Autodesk Inventor part; units mm, degrees
(part 2 of 3)
  arc A175 (-46.3689, 72.515) -> (-46.5311, 72.3209) centre (-45.3427, 71.4927) ccw
  line L41 (-46.5311, 72.3209) -> (-46.5959, 72.2278)
  line L42 (-46.5959, 72.2278) -> (-45.9786, 71.6449)
  line L43 (-45.9786, 71.6449) -> (-45.3612, 71.062)
  line L44 (-45.3612, 71.062) -> (-45.235, 71.2144)
  arc A176 (-44.7219, 71.7621) -> (-45.235, 71.2144) centre (-40.503, 67.2955) ccw
  arc A177 (-44.1577, 72.2287) -> (-44.7219, 71.7621) centre (-40.8999, 67.7158) ccw
  arc A178 (-43.5459, 72.611) -> (-44.1577, 72.2287) centre (-40.9969, 67.8501) ccw
  arc A179 (-42.8903, 72.907) -> (-43.5459, 72.611) centre (-41.0276, 67.9074) ccw
  arc A180 (-41.2076, 73.2541) -> (-42.8903, 72.907) centre (-40.9253, 67.6328) ccw
  arc A181 (-39.5165, 73.0714) -> (-41.2076, 73.2541) centre (-40.9361, 67.8491) ccw
  arc A182 (-37.9591, 72.3712) -> (-39.5165, 73.0714) centre (-40.9482, 67.8045) ccw
  arc A183 (-36.6652, 71.2147) -> (-37.9591, 72.3712) centre (-41.1435, 67.5061) ccw
  line L45 (-36.6652, 71.2147) -> (-36.5393, 71.0627)
  line L46 (-36.5393, 71.0627) -> (-35.9223, 71.6459)
  line L47 (-35.9223, 71.6459) -> (-35.3053, 72.2292)
  line L48 (-35.3053, 72.2292) -> (-35.3698, 72.3216)
  arc A184 (-35.3698, 72.3216) -> (-35.4148, 72.3777) centre (-35.8109, 72.0138) ccw
  arc A185 (-35.4148, 72.3777) -> (-35.5379, 72.51) centre (-46.5034, 62.1891) ccw
  arc A186 (-35.5379, 72.51) -> (-35.6869, 72.6659) centre (-45.6213, 63.0194) ccw
  arc A187 (-35.6869, 72.6659) -> (-35.8513, 72.8332) centre (-49.5707, 59.1844) ccw
  arc A188 (-35.8513, 72.8332) -> (-36.3178, 73.2672) centre (-41.6997, 67.0149) ccw
  arc A189 (-36.3178, 73.2672) -> (-36.7902, 73.6373) centre (-40.5561, 68.3435) ccw
  arc A190 (-36.7902, 73.6373) -> (-37.294, 73.9616) centre (-40.5426, 68.3625) ccw
  arc A191 (-37.294, 73.9616) -> (-37.8545, 74.2582) centre (-41.3698, 66.9368) ccw
  arc A192 (-37.8545, 74.2582) -> (-38.4115, 74.496) centre (-40.8225, 68.0766) ccw
  arc A193 (-38.4115, 74.496) -> (-38.9986, 74.689) centre (-41.0253, 67.5365) ccw
  arc A194 (-38.9986, 74.689) -> (-39.6005, 74.8329) centre (-41.0306, 67.518) ccw
  arc A195 (-39.6005, 74.8329) -> (-40.2018, 74.9233) centre (-40.9339, 68.0123) ccw
  arc A196 (-40.2018, 74.9233) -> (-40.5238, 74.9445) centre (-40.629, 70.891) ccw
  arc A197 (-40.5238, 74.9445) -> (-40.9902, 74.9502) centre (-40.9642, 57.9715) ccw
  arc A198 (-40.9902, 74.9502) -> (-41.4524, 74.9433) centre (-40.9639, 57.7224) ccw
  arc A199 (-41.4524, 74.9433) -> (-41.7507, 74.9209) centre (-41.3609, 71.7201) ccw
  arc A200 (-41.2579, 72.1952) -> (-42.0544, 72.0566) centre (-40.7232, 66.7647) ccw
  arc A201 (-42.0544, 72.0566) -> (-42.777, 71.8059) centre (-40.9868, 67.8125) ccw
  arc A202 (-42.777, 71.8059) -> (-43.4305, 71.4395) centre (-41.064, 67.9846) ccw
  arc A203 (-43.4305, 71.4395) -> (-44.0216, 70.9563) centre (-40.8808, 67.7173) ccw
  arc A204 (-44.0216, 70.9563) -> (-44.2114, 70.7646) centre (-39.4249, 66.2158) ccw
  arc A205 (-44.2114, 70.7646) -> (-44.3924, 70.5661) centre (-39.5049, 66.2919) ccw
  arc A206 (-44.3924, 70.5661) -> (-44.5501, 70.3821) centre (-35.0685, 62.4121) ccw
  arc A207 (-44.5501, 70.3821) -> (-44.5689, 70.3304) centre (-44.4886, 70.3304) ccw
  arc A208 (-44.5689, 70.3304) -> (-44.5593, 70.3082) centre (-44.5383, 70.3304) ccw
  arc A209 (-44.5593, 70.3082) -> (-43.965, 69.7486) centre (1428.2979, 1633.9609) ccw
  arc A210 (-43.965, 69.7486) -> (-43.3785, 69.197) centre (709.8736, 870.6675) ccw
  arc A211 (-43.3785, 69.197) -> (-43.337, 69.1709) centre (-43.2914, 69.2897) ccw
  arc A212 (-43.337, 69.1709) -> (-43.3227, 69.1742) centre (-43.3323, 69.1832) ccw
  arc A213 (-43.3227, 69.1742) -> (-43.2796, 69.2215) centre (-44.5899, 70.3724) ccw
  arc A214 (-43.2796, 69.2215) -> (-43.2296, 69.2821) centre (-44.2462, 70.0705) ccw
  arc A215 (-43.2296, 69.2821) -> (-43.1747, 69.3557) centre (-45.1202, 70.7483) ccw
  arc A216 (-42.8453, 69.7346) -> (-43.1747, 69.3557) centre (-41.0102, 67.8065) ccw
  arc A217 (-42.4468, 70.05) -> (-42.8453, 69.7346) centre (-40.9199, 67.7116) ccw
  arc A218 (-41.9954, 70.2896) -> (-42.4468, 70.05) centre (-40.9017, 67.6837) ccw
  arc A219 (-41.5087, 70.4437) -> (-41.9954, 70.2896) centre (-40.9069, 67.6961) ccw
  arc A220 (-41.2232, 70.4813) -> (-41.5087, 70.4437) centre (-41.1431, 68.7745) ccw
  arc A221 (-40.8534, 70.4837) -> (-41.2232, 70.4813) centre (-41.0092, 65.9221) ccw
  arc A222 (-40.4843, 70.4561) -> (-40.8534, 70.4837) centre (-41.0093, 65.9186) ccw
  arc A223 (-40.2008, 70.399) -> (-40.4843, 70.4561) centre (-40.6834, 68.7357) ccw
  arc A224 (-39.7681, 70.2293) -> (-40.2008, 70.399) centre (-40.9106, 67.9526) ccw
  arc A225 (-39.3522, 69.9772) -> (-39.7681, 70.2293) centre (-41.1362, 67.5029) ccw
  arc A226 (-38.983, 69.6632) -> (-39.3522, 69.9772) centre (-41.1244, 67.5193) ccw
  arc A227 (-38.6894, 69.3092) -> (-38.983, 69.6632) centre (-40.7215, 67.9227) ccw
  arc A228 (-38.6894, 69.3092) -> (-38.6489, 69.2532) centre (-37.6233, 70.0366) ccw
  arc A229 (-38.6489, 69.2532) -> (-38.6109, 69.2074) centre (-38.0844, 69.6844) ccw
  arc A230 (-38.6109, 69.2074) -> (-38.5781, 69.1735) centre (-38.075, 69.6929) ccw
  arc A231 (-38.5781, 69.1735) -> (-38.5639, 69.1706) centre (-38.5687, 69.1832) ccw
  arc A232 (-38.5639, 69.1706) -> (-38.5237, 69.1957) centre (-38.6075, 69.285) ccw
  arc A233 (-38.5237, 69.1957) -> (-37.9358, 69.7477) centre (-850.002, 934.1296) ccw
  arc A234 (-37.9358, 69.7477) -> (-37.3402, 70.3074) centre (-1609.827, 1742.9056) ccw
  arc A235 (-37.3402, 70.3074) -> (-37.3309, 70.3289) centre (-37.3604, 70.3289) ccw
  arc A236 (-37.3309, 70.3289) -> (-37.3338, 70.3377) centre (-37.3457, 70.3289) ccw
  arc A237 (-37.3338, 70.3377) -> (-37.376, 70.3946) centre (-47.3292, 62.9655) ccw
  arc A238 (-37.376, 70.3946) -> (-37.4256, 70.4597) centre (-40.8459, 67.8046) ccw
  arc A239 (-37.4256, 70.4597) -> (-37.4844, 70.5345) centre (-43.6707, 65.6119) ccw
  arc A240 (-37.4844, 70.5345) -> (-37.79, 70.8727) centre (-40.3313, 68.2691) ccw
  arc A241 (-37.79, 70.8727) -> (-38.1676, 71.2088) centre (-41.6249, 66.9438) ccw
  arc A242 (-38.1676, 71.2088) -> (-38.5756, 71.5096) centre (-41.641, 66.9241) ccw
  arc A243 (-38.5756, 71.5096) -> (-38.9731, 71.7413) centre (-40.6602, 68.3913) ccw
  arc A244 (-38.9731, 71.7413) -> (-39.2289, 71.8543) centre (-40.2179, 69.2696) ccw
  arc A245 (-39.2289, 71.8543) -> (-39.5614, 71.9719) centre (-41.6999, 65.3962) ccw
  arc A246 (-39.5614, 71.9719) -> (-39.9011, 72.0729) centre (-41.7094, 65.3668) ccw
  arc A247 (-39.9011, 72.0729) -> (-40.1799, 72.1338) centre (-40.6703, 69.2201) ccw
  arc A248 (-40.1799, 72.1338) -> (-40.4304, 72.1665) centre (-40.7514, 68.7389) ccw
  arc A249 (-40.4304, 72.1665) -> (-40.7499, 72.1906) centre (-41.2496, 63.417) ccw
  arc A250 (-40.7499, 72.1906) -> (-41.0583, 72.2028) centre (-41.2542, 63.3377) ccw
  arc A251 (-41.0583, 72.2028) -> (-41.2579, 72.1952) centre (-41.095, 70.5405) ccw
  arc A252 (-41.3041, 69.3977) -> (-41.7203, 69.2048) centre (-40.9224, 68.0282) ccw
  arc A253 (-41.7203, 69.2048) -> (-42.057, 68.8883) centre (-40.8992, 67.9939) ccw
  arc A254 (-42.057, 68.8883) -> (-42.2759, 68.4855) centre (-40.9189, 68.0091) ccw
  arc A255 (-42.2759, 68.4855) -> (-42.351, 68.0425) centre (-41.0214, 68.0451) ccw
  arc A256 (-42.351, 68.0425) -> (-42.2073, 67.4314) centre (-40.9678, 68.0452) ccw
  arc A257 (-42.2073, 67.4314) -> (-41.8076, 66.9404) centre (-40.9266, 68.0656) ccw
  arc A258 (-41.8076, 66.9404) -> (-41.2375, 66.6724) centre (-40.937, 68.0524) ccw
  arc A259 (-41.2375, 66.6724) -> (-40.6171, 66.6849) centre (-40.9535, 67.9765) ccw
  arc A260 (-40.6171, 66.6849) -> (-40.2585, 66.8282) centre (-41.0066, 68.1804) ccw
  arc A261 (-40.2585, 66.8282) -> (-39.9614, 67.0519) centre (-40.9034, 67.9939) ccw
  arc A262 (-39.9614, 67.0519) -> (-39.7377, 67.3489) centre (-40.9034, 67.9939) ccw
  arc A263 (-39.7377, 67.3489) -> (-39.5945, 67.7075) centre (-41.0899, 68.0971) ccw
  arc A264 (-39.5945, 67.7075) -> (-39.5827, 68.335) centre (-40.8932, 68.0458) ccw
  arc A265 (-39.5827, 68.335) -> (-39.8564, 68.9075) centre (-40.949, 68.0335) ccw
  arc A266 (-39.8564, 68.9075) -> (-40.3572, 69.3039) centre (-40.9658, 68.02) ccw
  arc A267 (-40.3572, 69.3039) -> (-40.9795, 69.439) centre (-40.9587, 68.0351) ccw
  arc A268 (-40.9795, 69.439) -> (-41.0608, 69.4352) centre (-40.9611, 68.1934) ccw
  arc A269 (-41.0608, 69.4352) -> (-41.1516, 69.4257) centre (-40.904, 67.4834) ccw
  arc A270 (-41.1516, 69.4257) -> (-41.2378, 69.4127) centre (-40.9176, 67.5898) ccw
  arc A271 (-41.2378, 69.4127) -> (-41.3041, 69.3977) centre (-41.1176, 68.7282) ccw
  arc A272 (-54.2587, 71.8195) -> (-55.2164, 71.6633) centre (-53.721, 65.5053) ccw
  arc A273 (-55.2164, 71.6633) -> (-56.1281, 71.3638) centre (-53.7854, 65.7705) ccw
  arc A274 (-56.1281, 71.3638) -> (-56.9803, 70.9245) centre (-53.7898, 65.7811) ccw
  arc A275 (-56.9803, 70.9245) -> (-57.761, 70.3525) centre (-53.6689, 65.5862) ccw
  arc A276 (-57.761, 70.3525) -> (-57.9303, 70.1998) centre (-54.7143, 66.8038) ccw
  arc A277 (-57.9303, 70.1998) -> (-58.1244, 70.0106) centre (-51.5447, 63.4568) ccw
  arc A278 (-58.1244, 70.0106) -> (-58.3037, 69.8254) centre (-51.7023, 63.6139) ccw
  arc A279 (-58.3037, 69.8254) -> (-58.4189, 69.6921) centre (-56.7958, 68.4066) ccw
  line L49 (-58.4189, 69.6921) -> (-58.4764, 69.6194)
  line L50 (-58.4764, 69.6194) -> (-58.0951, 69.2684)
  line L51 (-58.0951, 69.2684) -> (-57.7138, 68.9174)
  line L52 (-57.7138, 68.9174) -> (-57.6118, 69.0338)
  arc A280 (-57.0139, 69.616) -> (-57.6118, 69.0338) centre (-53.6679, 65.5813) ccw
  arc A281 (-56.3308, 70.0963) -> (-57.0139, 69.616) centre (-53.6618, 65.5739) ccw
  arc A282 (-55.5869, 70.4582) -> (-56.3308, 70.0963) centre (-53.7111, 65.6576) ccw
  arc A283 (-54.8079, 70.6887) -> (-55.5869, 70.4582) centre (-53.8421, 65.9928) ccw
  arc A284 (-54.2943, 70.7669) -> (-54.8079, 70.6887) centre (-53.7974, 65.7752) ccw
  arc A285 (-53.7678, 70.793) -> (-54.2943, 70.7669) centre (-53.7678, 65.4777) ccw
  arc A286 (-53.2413, 70.7669) -> (-53.7678, 70.793) centre (-53.7678, 65.4777) ccw
  arc A287 (-52.7277, 70.6887) -> (-53.2413, 70.7669) centre (-53.7382, 65.7752) ccw
  arc A288 (-51.9486, 70.4585) -> (-52.7277, 70.6887) centre (-53.6976, 65.9726) ccw
  arc A289 (-51.2067, 70.0979) -> (-51.9486, 70.4585) centre (-53.8074, 65.6909) ccw
  arc A290 (-50.5247, 69.6182) -> (-51.2067, 70.0979) centre (-53.8645, 65.5942) ccw
  arc A291 (-49.9239, 69.034) -> (-50.5247, 69.6182) centre (-53.9323, 65.5125) ccw
  line L53 (-49.9239, 69.034) -> (-49.8218, 68.9178)
  line L54 (-49.8218, 68.9178) -> (-49.4403, 69.2684)
  line L55 (-49.4403, 69.2684) -> (-49.0588, 69.619)
  line L56 (-49.0588, 69.619) -> (-49.1187, 69.6961)
  arc A292 (-49.1187, 69.6961) -> (-49.2435, 69.8387) centre (-50.3783, 68.7188) ccw
  arc A293 (-49.2435, 69.8387) -> (-49.4908, 70.0838) centre (-60.4502, 58.7794) ccw
  arc A294 (-49.4908, 70.0838) -> (-49.7488, 70.3278) centre (-59.4752, 59.7852) ccw
  arc A295 (-49.7488, 70.3278) -> (-49.9351, 70.4876) centre (-52.0641, 67.8182) ccw
  arc A296 (-49.9351, 70.4876) -> (-50.698, 71.0097) centre (-53.8793, 65.5422) ccw
  arc A297 (-50.698, 71.0097) -> (-51.5212, 71.4089) centre (-53.7491, 65.766) ccw
  arc A298 (-51.5212, 71.4089) -> (-52.3959, 71.6801) centre (-53.7544, 65.7527) ccw
  arc A299 (-52.3959, 71.6801) -> (-53.3127, 71.8212) centre (-53.8245, 65.4466) ccw
  arc A300 (-53.3127, 71.8212) -> (-53.5357, 71.8337) centre (-53.6841, 67.195) ccw
  arc A301 (-53.5357, 71.8337) -> (-53.7872, 71.8375) centre (-53.7737, 64.3958) ccw
  arc A302 (-53.7872, 71.8375) -> (-54.0379, 71.8328) centre (-53.7737, 64.4287) ccw
  arc A303 (-54.0379, 71.8328) -> (-54.2587, 71.8195) centre (-53.8779, 67.3479) ccw
  arc A304 (-54.2587, 70.1206) -> (-54.8466, 70.011) centre (-53.685, 65.4098) ccw
  arc A305 (-54.8466, 70.011) -> (-55.4044, 69.8298) centre (-53.7721, 65.755) ccw
  arc A306 (-55.4044, 69.8298) -> (-55.9344, 69.5753) centre (-53.7639, 65.7344) ccw
  arc A307 (-55.9344, 69.5753) -> (-56.4394, 69.2471) centre (-53.5452, 65.3475) ccw
  arc A308 (-56.4394, 69.2471) -> (-56.6021, 69.1131) centre (-55.1906, 67.5645) ccw
  arc A309 (-56.6021, 69.1131) -> (-56.8494, 68.8817) centre (-47.9272, 59.5958) ccw
  arc A310 (-56.8494, 68.8817) -> (-57.0896, 68.6458) centre (-46.1793, 57.7765) ccw
  arc A311 (-57.0896, 68.6458) -> (-57.189, 68.5268) centre (-56.4605, 68.0191) ccw
  line L57 (-57.189, 68.5268) -> (-57.2288, 68.4697)
  line L58 (-57.2288, 68.4697) -> (-56.8503, 68.1124)
  line L59 (-56.8503, 68.1124) -> (-56.4719, 67.7551)
  line L60 (-56.4719, 67.7551) -> (-56.3945, 67.8485)
  arc A312 (-56.08, 68.1842) -> (-56.3945, 67.8485) centre (-53.4938, 65.4462) ccw
  arc A313 (-55.7342, 68.4703) -> (-56.08, 68.1842) centre (-53.7371, 65.7039) ccw
  arc A314 (-55.3591, 68.7046) -> (-55.7342, 68.4703) centre (-53.7966, 65.7862) ccw
  arc A315 (-54.9572, 68.886) -> (-55.3591, 68.7046) centre (-53.8154, 65.8213) ccw
  arc A316 (-53.9257, 69.0988) -> (-54.9572, 68.886) centre (-53.7527, 65.653) ccw
  arc A317 (-52.8891, 68.9868) -> (-53.9257, 69.0988) centre (-53.7593, 65.7856) ccw
  arc A318 (-51.9344, 68.5576) -> (-52.8891, 68.9868) centre (-53.7667, 65.7582) ccw
  arc A319 (-51.1412, 67.8487) -> (-51.9344, 68.5576) centre (-53.8865, 65.5753) ccw
  line L61 (-51.1412, 67.8487) -> (-51.064, 67.7555)
  line L62 (-51.064, 67.7555) -> (-50.6858, 68.113)
  line L63 (-50.6858, 68.113) -> (-50.3077, 68.4706)
  line L64 (-50.3077, 68.4706) -> (-50.3472, 68.5272)
  arc A320 (-50.3472, 68.5272) -> (-50.3748, 68.5616) centre (-50.6176, 68.3385) ccw
  arc A321 (-50.3748, 68.5616) -> (-50.4502, 68.6427) centre (-57.1721, 62.316) ccw
  arc A322 (-50.4502, 68.6427) -> (-50.5416, 68.7383) centre (-56.6313, 62.825) ccw
  arc A323 (-50.5416, 68.7383) -> (-50.6423, 68.8408) centre (-59.0523, 60.4741) ccw
  arc A324 (-50.6423, 68.8408) -> (-50.9283, 69.1069) centre (-54.2274, 65.2742) ccw
  arc A325 (-50.9283, 69.1069) -> (-51.2179, 69.3337) centre (-53.5264, 66.0886) ccw
  arc A326 (-51.2179, 69.3337) -> (-51.5267, 69.5325) centre (-53.5181, 66.1003) ccw
  arc A327 (-51.5267, 69.5325) -> (-51.8703, 69.7143) centre (-54.0251, 65.2263) ccw
  arc A328 (-51.8703, 69.7143) -> (-52.2117, 69.8601) centre (-53.6897, 65.9251) ccw
  arc A329 (-52.2117, 69.8601) -> (-52.5716, 69.9784) centre (-53.814, 65.594) ccw
  arc A330 (-52.5716, 69.9784) -> (-52.9406, 70.0666) centre (-53.8172, 65.5826) ccw
  arc A331 (-52.9406, 70.0666) -> (-53.3092, 70.1221) centre (-53.758, 65.8856) ccw
  arc A332 (-53.3092, 70.1221) -> (-53.5066, 70.1351) centre (-53.571, 67.6502) ccw
  arc A333 (-53.5066, 70.1351) -> (-53.7925, 70.1386) centre (-53.7766, 59.7306) ccw
  arc A334 (-53.7925, 70.1386) -> (-54.0758, 70.1343) centre (-53.7763, 59.5779) ccw
  arc A335 (-54.0758, 70.1343) -> (-54.2587, 70.1206) centre (-54.0197, 68.1585) ccw
  arc A336 (-53.9566, 68.4497) -> (-54.4448, 68.3648) centre (-53.6288, 65.1208) ccw
  arc A337 (-54.4448, 68.3648) -> (-54.8878, 68.2111) centre (-53.7904, 65.7631) ccw
  arc A338 (-54.8878, 68.2111) -> (-55.2884, 67.9865) centre (-53.8377, 65.8687) ccw
  arc A339 (-55.2884, 67.9865) -> (-55.6507, 67.6903) centre (-53.7254, 65.7048) ccw
  arc A340 (-55.6507, 67.6903) -> (-55.7671, 67.5728) centre (-52.8329, 64.7844) ccw
  arc A341 (-55.7671, 67.5728) -> (-55.878, 67.4511) centre (-52.882, 64.831) ccw
  arc A342 (-55.878, 67.4511) -> (-55.9747, 67.3383) centre (-50.1625, 62.4527) ccw
  arc A343 (-55.9747, 67.3383) -> (-55.9862, 67.3066) centre (-55.937, 67.3066) ccw
  arc A344 (-55.9862, 67.3066) -> (-55.9803, 67.293) centre (-55.9675, 67.3066) ccw
  arc A345 (-55.9803, 67.293) -> (-55.616, 66.95) centre (846.8811, 1025.8121) ccw
  arc A346 (-55.616, 66.95) -> (-55.2565, 66.6118) centre (406.487, 557.9133) ccw
  arc A347 (-55.2565, 66.6118) -> (-55.2311, 66.5959) centre (-55.2031, 66.6687) ccw
  arc A348 (-55.2311, 66.5959) -> (-55.2223, 66.5979) centre (-55.2282, 66.6034) ccw
  arc A349 (-55.2223, 66.5979) -> (-55.1959, 66.6269) centre (-55.9991, 67.3324) ccw
  arc A350 (-55.1959, 66.6269) -> (-55.1652, 66.664) centre (-55.7884, 67.1473) ccw
  arc A351 (-55.1652, 66.664) -> (-55.1316, 66.7092) centre (-56.3242, 67.5628) ccw
  arc A352 (-54.9296, 66.9414) -> (-55.1316, 66.7092) centre (-53.8047, 65.7595) ccw
  arc A353 (-54.6854, 67.1347) -> (-54.9296, 66.9414) centre (-53.7494, 65.7013) ccw
  arc A354 (-54.4086, 67.2816) -> (-54.6854, 67.1347) centre (-53.7382, 65.6842) ccw
  arc A355 (-54.1103, 67.376) -> (-54.4086, 67.2816) centre (-53.7414, 65.6918) ccw
  arc A356 (-53.9353, 67.3991) -> (-54.1103, 67.376) centre (-53.8862, 66.3529) ccw
  arc A357 (-53.7086, 67.4006) -> (-53.9353, 67.3991) centre (-53.8041, 64.6043) ccw
  arc A358 (-53.4824, 67.3837) -> (-53.7086, 67.4006) centre (-53.8042, 64.6022) ccw
  arc A359 (-53.3086, 67.3487) -> (-53.4824, 67.3837) centre (-53.6044, 66.3291) ccw
  arc A360 (-53.0433, 67.2446) -> (-53.3086, 67.3487) centre (-53.7437, 65.849) ccw
  arc A361 (-52.7884, 67.0901) -> (-53.0433, 67.2446) centre (-53.882, 65.5734) ccw
  arc A362 (-52.562, 66.8976) -> (-52.7884, 67.0901) centre (-53.8748, 65.5834) ccw
  arc A363 (-52.3821, 66.6806) -> (-52.562, 66.8976) centre (-53.6278, 65.8307) ccw
  arc A364 (-52.3821, 66.6806) -> (-52.3573, 66.6463) centre (-51.7286, 67.1265) ccw
  arc A365 (-52.3573, 66.6463) -> (-52.3339, 66.6182) centre (-52.0112, 66.9106) ccw
  arc A366 (-52.3339, 66.6182) -> (-52.3138, 66.5974) centre (-52.0055, 66.9158) ccw
  arc A367 (-52.3138, 66.5974) -> (-52.3051, 66.5957) centre (-52.3081, 66.6034) ccw
  arc A368 (-52.3051, 66.5957) -> (-52.2805, 66.611) centre (-52.3319, 66.6658) ccw
  arc A369 (-52.2805, 66.611) -> (-51.9201, 66.9494) centre (-549.7167, 596.8155) ccw
  arc A370 (-51.9201, 66.9494) -> (-51.555, 67.2925) centre (-1015.4894, 1092.5952) ccw
  arc A371 (-51.555, 67.2925) -> (-51.5493, 67.3057) centre (-51.5674, 67.3057) ccw
  arc A372 (-51.5493, 67.3057) -> (-51.5511, 67.3111) centre (-51.5584, 67.3057) ccw
  arc A373 (-51.5511, 67.3111) -> (-51.577, 67.3459) centre (-57.6783, 62.7919) ccw
  arc A374 (-51.577, 67.3459) -> (-51.6073, 67.3859) centre (-53.704, 65.7583) ccw
  arc A375 (-51.6073, 67.3859) -> (-51.6434, 67.4317) centre (-55.4356, 64.4141) ccw
  arc A376 (-51.6434, 67.4317) -> (-51.8307, 67.6391) centre (-53.3886, 66.043) ccw
  arc A377 (-51.8307, 67.6391) -> (-52.0622, 67.8451) centre (-54.1816, 65.2306) ccw
  arc A378 (-52.0622, 67.8451) -> (-52.3124, 68.0294) centre (-54.1914, 65.2185) ccw
  arc A379 (-52.3124, 68.0294) -> (-52.556, 68.1715) centre (-53.5902, 66.1179) ccw
  arc A380 (-52.556, 68.1715) -> (-52.7128, 68.2408) centre (-53.319, 66.6563) ccw
  arc A381 (-52.7128, 68.2408) -> (-52.9166, 68.3129) centre (-54.2275, 64.282) ccw
  arc A382 (-52.9166, 68.3129) -> (-53.1248, 68.3747) centre (-54.2334, 64.2639) ccw
  arc A383 (-53.1248, 68.3747) -> (-53.2958, 68.4121) centre (-53.5964, 66.626) ccw
  arc A384 (-53.2958, 68.4121) -> (-53.4493, 68.4322) centre (-53.6461, 66.331) ccw
  arc A385 (-53.4493, 68.4322) -> (-53.6452, 68.4469) centre (-53.9515, 63.0687) ccw
  arc A386 (-53.6452, 68.4469) -> (-53.8342, 68.4544) centre (-53.9543, 63.0201) ccw
  arc A387 (-53.8342, 68.4544) -> (-53.9566, 68.4497) centre (-53.8567, 67.4354) ccw
  arc A388 (-53.9849, 66.7348) -> (-54.24, 66.6166) centre (-53.7509, 65.8954) ccw
  arc A389 (-54.24, 66.6166) -> (-54.4464, 66.4226) centre (-53.7367, 65.8744) ccw
  arc A390 (-54.4464, 66.4226) -> (-54.5806, 66.1757) centre (-53.7487, 65.8837) ccw
  arc A391 (-54.5806, 66.1757) -> (-54.6266, 65.9041) centre (-53.8116, 65.9057) ccw
  arc A392 (-54.6266, 65.9041) -> (-54.5386, 65.5295) centre (-53.7788, 65.9058) ccw
  arc A393 (-54.5386, 65.5295) -> (-54.2936, 65.2285) centre (-53.7535, 65.9183) ccw
  arc A394 (-54.2936, 65.2285) -> (-53.9441, 65.0643) centre (-53.7598, 65.9102) ccw
  arc A395 (-53.9441, 65.0643) -> (-53.5637, 65.0719) centre (-53.77, 65.8637) ccw
  arc A396 (-53.5637, 65.0719) -> (-53.3439, 65.1598) centre (-53.8025, 65.9887) ccw
  arc A397 (-53.3439, 65.1598) -> (-53.1618, 65.2969) centre (-53.7393, 65.8743) ccw
  arc A398 (-53.1618, 65.2969) -> (-53.0247, 65.479) centre (-53.7393, 65.8743) ccw
  arc A399 (-53.0247, 65.479) -> (-52.9369, 65.6988) centre (-53.8536, 65.9376) ccw
  arc A400 (-52.9369, 65.6988) -> (-52.9297, 66.0834) centre (-53.733, 65.9062) ccw
  arc A401 (-52.9297, 66.0834) -> (-53.0974, 66.4344) centre (-53.7672, 65.8986) ccw
  arc A402 (-53.0974, 66.4344) -> (-53.4045, 66.6773) centre (-53.7775, 65.8904) ccw
  arc A403 (-53.4045, 66.6773) -> (-53.7859, 66.7602) centre (-53.7732, 65.8996) ccw
  arc A404 (-53.7859, 66.7602) -> (-53.8358, 66.7578) centre (-53.7746, 65.9967) ccw
  arc A405 (-53.8358, 66.7578) -> (-53.8914, 66.7521) centre (-53.7396, 65.5614) ccw
  arc A406 (-53.8914, 66.7521) -> (-53.9443, 66.7441) centre (-53.7479, 65.6266) ccw
  arc A407 (-53.9443, 66.7441) -> (-53.9849, 66.7348) centre (-53.8705, 66.3245) ccw
  arc A408 (-9.2413, 17.0805) -> (-8.2836, 17.2367) centre (-9.779, 23.3947) ccw
  arc A409 (-8.2836, 17.2367) -> (-7.3719, 17.5362) centre (-9.7146, 23.1295) ccw
  arc A410 (-7.3719, 17.5362) -> (-6.5197, 17.9755) centre (-9.7102, 23.1189) ccw
  arc A411 (-6.5197, 17.9755) -> (-5.739, 18.5475) centre (-9.8311, 23.3138) ccw
  arc A412 (-5.739, 18.5475) -> (-5.5697, 18.7002) centre (-8.7857, 22.0962) ccw
  arc A413 (-5.5697, 18.7002) -> (-5.3756, 18.8894) centre (-11.9553, 25.4432) ccw
  arc A414 (-5.3756, 18.8894) -> (-5.1963, 19.0746) centre (-11.7977, 25.2861) ccw
  arc A415 (-5.1963, 19.0746) -> (-5.0811, 19.2079) centre (-6.7042, 20.4934) ccw
  line L65 (-5.0811, 19.2079) -> (-5.0236, 19.2806)
  line L66 (-5.0236, 19.2806) -> (-5.4049, 19.6316)
  line L67 (-5.4049, 19.6316) -> (-5.7862, 19.9826)
  line L68 (-5.7862, 19.9826) -> (-5.8882, 19.8662)
  arc A416 (-6.4861, 19.284) -> (-5.8882, 19.8662) centre (-9.8321, 23.3187) ccw
  arc A417 (-7.1692, 18.8037) -> (-6.4861, 19.284) centre (-9.8382, 23.3261) ccw
  arc A418 (-7.9131, 18.4418) -> (-7.1692, 18.8037) centre (-9.7889, 23.2424) ccw
  arc A419 (-8.6921, 18.2113) -> (-7.9131, 18.4418) centre (-9.6579, 22.9072) ccw
  arc A420 (-9.2057, 18.1331) -> (-8.6921, 18.2113) centre (-9.7026, 23.1248) ccw
  arc A421 (-9.7322, 18.107) -> (-9.2057, 18.1331) centre (-9.7322, 23.4223) ccw
  arc A422 (-10.2587, 18.1331) -> (-9.7322, 18.107) centre (-9.7322, 23.4223) ccw
  arc A423 (-10.7723, 18.2113) -> (-10.2587, 18.1331) centre (-9.7618, 23.1248) ccw
  arc A424 (-11.5514, 18.4415) -> (-10.7723, 18.2113) centre (-9.8024, 22.9274) ccw
  arc A425 (-12.2933, 18.8021) -> (-11.5514, 18.4415) centre (-9.6926, 23.2091) ccw
  arc A426 (-12.9753, 19.2818) -> (-12.2933, 18.8021) centre (-9.6355, 23.3058) ccw
  arc A427 (-13.5761, 19.866) -> (-12.9753, 19.2818) centre (-9.5677, 23.3875) ccw
  line L69 (-13.5761, 19.866) -> (-13.6782, 19.9822)
  line L70 (-13.6782, 19.9822) -> (-14.0597, 19.6316)
  line L71 (-14.0597, 19.6316) -> (-14.4412, 19.281)
  line L72 (-14.4412, 19.281) -> (-14.3813, 19.2039)
  arc A428 (-14.3813, 19.2039) -> (-14.2565, 19.0613) centre (-13.1217, 20.1812) ccw
  arc A429 (-14.2565, 19.0613) -> (-14.0092, 18.8162) centre (-3.0498, 30.1206) ccw
  arc A430 (-14.0092, 18.8162) -> (-13.7512, 18.5722) centre (-4.0248, 29.1148) ccw
  arc A431 (-13.7512, 18.5722) -> (-13.5649, 18.4124) centre (-11.4359, 21.0818) ccw
  arc A432 (-13.5649, 18.4124) -> (-12.802, 17.8903) centre (-9.6207, 23.3578) ccw
  arc A433 (-12.802, 17.8903) -> (-11.9788, 17.4911) centre (-9.7509, 23.134) ccw
  arc A434 (-11.9788, 17.4911) -> (-11.1041, 17.2199) centre (-9.7456, 23.1473) ccw
  arc A435 (-11.1041, 17.2199) -> (-10.1873, 17.0788) centre (-9.6755, 23.4534) ccw
  arc A436 (-10.1873, 17.0788) -> (-9.9643, 17.0663) centre (-9.8159, 21.705) ccw
  arc A437 (-9.9643, 17.0663) -> (-9.7128, 17.0625) centre (-9.7263, 24.5042) ccw
  arc A438 (-9.7128, 17.0625) -> (-9.4621, 17.0672) centre (-9.7263, 24.4713) ccw
  arc A439 (-9.4621, 17.0672) -> (-9.2413, 17.0805) centre (-9.6221, 21.5521) ccw
  arc A440 (-9.2413, 18.7794) -> (-8.6534, 18.889) centre (-9.815, 23.4902) ccw
  arc A441 (-8.6534, 18.889) -> (-8.0956, 19.0702) centre (-9.7279, 23.145) ccw
  arc A442 (-8.0956, 19.0702) -> (-7.5656, 19.3247) centre (-9.7361, 23.1656) ccw
  arc A443 (-7.5656, 19.3247) -> (-7.0606, 19.6529) centre (-9.9548, 23.5525) ccw
  arc A444 (-7.0606, 19.6529) -> (-6.8979, 19.7869) centre (-8.3094, 21.3355) ccw
  arc A445 (-6.8979, 19.7869) -> (-6.6506, 20.0183) centre (-15.5728, 29.3042) ccw
  arc A446 (-6.6506, 20.0183) -> (-6.4104, 20.2542) centre (-17.3207, 31.1235) ccw
  arc A447 (-6.4104, 20.2542) -> (-6.311, 20.3732) centre (-7.0395, 20.8809) ccw
  line L73 (-6.311, 20.3732) -> (-6.2712, 20.4303)
  line L74 (-6.2712, 20.4303) -> (-6.6497, 20.7876)
  line L75 (-6.6497, 20.7876) -> (-7.0281, 21.1449)
  line L76 (-7.0281, 21.1449) -> (-7.1055, 21.0515)
  arc A448 (-7.42, 20.7158) -> (-7.1055, 21.0515) centre (-10.0062, 23.4538) ccw
  arc A449 (-7.7658, 20.4297) -> (-7.42, 20.7158) centre (-9.7629, 23.1961) ccw
  arc A450 (-8.1409, 20.1954) -> (-7.7658, 20.4297) centre (-9.7034, 23.1138) ccw
  arc A451 (-8.5428, 20.014) -> (-8.1409, 20.1954) centre (-9.6846, 23.0787) ccw
  arc A452 (-9.5743, 19.8012) -> (-8.5428, 20.014) centre (-9.7473, 23.247) ccw
  arc A453 (-10.6109, 19.9132) -> (-9.5743, 19.8012) centre (-9.7407, 23.1144) ccw
  arc A454 (-11.5656, 20.3424) -> (-10.6109, 19.9132) centre (-9.7333, 23.1418) ccw
  arc A455 (-12.3588, 21.0513) -> (-11.5656, 20.3424) centre (-9.6135, 23.3247) ccw
  line L77 (-12.3588, 21.0513) -> (-12.436, 21.1445)
  line L78 (-12.436, 21.1445) -> (-12.8142, 20.787)
  line L79 (-12.8142, 20.787) -> (-13.1923, 20.4294)
  line L80 (-13.1923, 20.4294) -> (-13.1528, 20.3728)
  arc A456 (-13.1528, 20.3728) -> (-13.1252, 20.3384) centre (-12.8824, 20.5615) ccw
  arc A457 (-13.1252, 20.3384) -> (-13.0498, 20.2573) centre (-6.3279, 26.584) ccw
  arc A458 (-13.0498, 20.2573) -> (-12.9584, 20.1617) centre (-6.8687, 26.075) ccw
  arc A459 (-12.9584, 20.1617) -> (-12.8577, 20.0592) centre (-4.4477, 28.4259) ccw
  arc A460 (-12.8577, 20.0592) -> (-12.5717, 19.7931) centre (-9.2726, 23.6258) ccw
  arc A461 (-12.5717, 19.7931) -> (-12.2821, 19.5663) centre (-9.9736, 22.8114) ccw
  arc A462 (-12.2821, 19.5663) -> (-11.9733, 19.3675) centre (-9.9819, 22.7997) ccw
  arc A463 (-11.9733, 19.3675) -> (-11.6297, 19.1857) centre (-9.4749, 23.6737) ccw
  arc A464 (-11.6297, 19.1857) -> (-11.2883, 19.0399) centre (-9.8103, 22.9749) ccw
  arc A465 (-11.2883, 19.0399) -> (-10.9284, 18.9216) centre (-9.686, 23.306) ccw
  arc A466 (-10.9284, 18.9216) -> (-10.5594, 18.8334) centre (-9.6828, 23.3174) ccw
  arc A467 (-10.5594, 18.8334) -> (-10.1908, 18.7779) centre (-9.742, 23.0144) ccw
  arc A468 (-10.1908, 18.7779) -> (-9.9934, 18.7649) centre (-9.929, 21.2498) ccw
  arc A469 (-9.9934, 18.7649) -> (-9.7075, 18.7614) centre (-9.7234, 29.1694) ccw
  arc A470 (-9.7075, 18.7614) -> (-9.4242, 18.7657) centre (-9.7237, 29.3221) ccw
  arc A471 (-9.4242, 18.7657) -> (-9.2413, 18.7794) centre (-9.4803, 20.7415) ccw
  arc A472 (-9.5434, 20.4503) -> (-9.0552, 20.5352) centre (-9.8712, 23.7792) ccw
  arc A473 (-9.0552, 20.5352) -> (-8.6122, 20.6889) centre (-9.7096, 23.1369) ccw
  arc A474 (-8.6122, 20.6889) -> (-8.2116, 20.9135) centre (-9.6623, 23.0313) ccw
  arc A475 (-8.2116, 20.9135) -> (-7.8493, 21.2097) centre (-9.7746, 23.1952) ccw
  arc A476 (-7.8493, 21.2097) -> (-7.7329, 21.3272) centre (-10.6671, 24.1156) ccw
  arc A477 (-7.7329, 21.3272) -> (-7.622, 21.4489) centre (-10.618, 24.069) ccw
  arc A478 (-7.622, 21.4489) -> (-7.5253, 21.5617) centre (-13.3375, 26.4473) ccw
  arc A479 (-7.5253, 21.5617) -> (-7.5138, 21.5934) centre (-7.563, 21.5934) ccw
  arc A480 (-7.5138, 21.5934) -> (-7.5197, 21.607) centre (-7.5325, 21.5934) ccw
  arc A481 (-7.5197, 21.607) -> (-7.884, 21.95) centre (-910.3811, -936.9121) ccw
  arc A482 (-7.884, 21.95) -> (-8.2435, 22.2882) centre (-469.987, -469.0133) ccw
  arc A483 (-8.2435, 22.2882) -> (-8.2689, 22.3041) centre (-8.2969, 22.2313) ccw
  arc A484 (-8.2689, 22.3041) -> (-8.2777, 22.3021) centre (-8.2718, 22.2966) ccw
  arc A485 (-8.2777, 22.3021) -> (-8.3041, 22.2731) centre (-7.5009, 21.5676) ccw
  arc A486 (-8.3041, 22.2731) -> (-8.3348, 22.236) centre (-7.7116, 21.7527) ccw
  arc A487 (-8.3348, 22.236) -> (-8.3684, 22.1908) centre (-7.1758, 21.3372) ccw
  arc A488 (-8.5704, 21.9586) -> (-8.3684, 22.1908) centre (-9.6953, 23.1405) ccw
  arc A489 (-8.8146, 21.7653) -> (-8.5704, 21.9586) centre (-9.7506, 23.1987) ccw
  arc A490 (-9.0914, 21.6184) -> (-8.8146, 21.7653) centre (-9.7618, 23.2158) ccw
  arc A491 (-9.3897, 21.524) -> (-9.0914, 21.6184) centre (-9.7586, 23.2082) ccw
  arc A492 (-9.5647, 21.5009) -> (-9.3897, 21.524) centre (-9.6138, 22.5471) ccw
  arc A493 (-9.7914, 21.4994) -> (-9.5647, 21.5009) centre (-9.6959, 24.2957) ccw
  arc A494 (-10.0176, 21.5163) -> (-9.7914, 21.4994) centre (-9.6958, 24.2978) ccw
  arc A495 (-10.1914, 21.5513) -> (-10.0176, 21.5163) centre (-9.8956, 22.5709) ccw
  arc A496 (-10.4567, 21.6554) -> (-10.1914, 21.5513) centre (-9.7563, 23.051) ccw
  arc A497 (-10.7116, 21.8099) -> (-10.4567, 21.6554) centre (-9.618, 23.3266) ccw
  arc A498 (-10.938, 22.0024) -> (-10.7116, 21.8099) centre (-9.6252, 23.3166) ccw
  arc A499 (-11.1179, 22.2194) -> (-10.938, 22.0024) centre (-9.8722, 23.0693) ccw
  arc A500 (-11.1179, 22.2194) -> (-11.1427, 22.2537) centre (-11.7714, 21.7735) ccw
  arc A501 (-11.1427, 22.2537) -> (-11.1661, 22.2818) centre (-11.4888, 21.9894) ccw
  arc A502 (-11.1661, 22.2818) -> (-11.1862, 22.3026) centre (-11.4945, 21.9842) ccw
  arc A503 (-11.1862, 22.3026) -> (-11.1949, 22.3043) centre (-11.1919, 22.2966) ccw
  arc A504 (-11.1949, 22.3043) -> (-11.2195, 22.289) centre (-11.1681, 22.2342) ccw
  arc A505 (-11.2195, 22.289) -> (-11.5799, 21.9506) centre (486.2167, -507.9155) ccw
  arc A506 (-11.5799, 21.9506) -> (-11.945, 21.6075) centre (951.9894, -1003.6952) ccw
  arc A507 (-11.945, 21.6075) -> (-11.9507, 21.5943) centre (-11.9326, 21.5943) ccw
  arc A508 (-11.9507, 21.5943) -> (-11.9489, 21.5889) centre (-11.9416, 21.5943) ccw
  arc A509 (-11.9489, 21.5889) -> (-11.923, 21.5541) centre (-5.8217, 26.1081) ccw
  arc A510 (-11.923, 21.5541) -> (-11.8927, 21.5141) centre (-9.796, 23.1417) ccw
  arc A511 (-11.8927, 21.5141) -> (-11.8566, 21.4683) centre (-8.0644, 24.4859) ccw
  arc A512 (-11.8566, 21.4683) -> (-11.6693, 21.2609) centre (-10.1114, 22.857) ccw
  arc A513 (-11.6693, 21.2609) -> (-11.4378, 21.0549) centre (-9.3184, 23.6694) ccw
  arc A514 (-11.4378, 21.0549) -> (-11.1876, 20.8706) centre (-9.3086, 23.6815) ccw
  arc A515 (-11.1876, 20.8706) -> (-10.944, 20.7285) centre (-9.9098, 22.7821) ccw
  arc A516 (-10.944, 20.7285) -> (-10.7872, 20.6592) centre (-10.181, 22.2437) ccw
  arc A517 (-10.7872, 20.6592) -> (-10.5834, 20.5871) centre (-9.2725, 24.618) ccw
  arc A518 (-10.5834, 20.5871) -> (-10.3752, 20.5253) centre (-9.2666, 24.6361) ccw
  arc A519 (-10.3752, 20.5253) -> (-10.2042, 20.4879) centre (-9.9036, 22.274) ccw
  arc A520 (-10.2042, 20.4879) -> (-10.0507, 20.4678) centre (-9.8539, 22.569) ccw
  arc A521 (-10.0507, 20.4678) -> (-9.8548, 20.4531) centre (-9.5485, 25.8313) ccw
  arc A522 (-9.8548, 20.4531) -> (-9.6658, 20.4456) centre (-9.5457, 25.8799) ccw
  arc A523 (-9.6658, 20.4456) -> (-9.5434, 20.4503) centre (-9.6433, 21.4646) ccw
  arc A524 (-9.5151, 22.1652) -> (-9.26, 22.2834) centre (-9.7491, 23.0046) ccw
  arc A525 (-9.26, 22.2834) -> (-9.0536, 22.4774) centre (-9.7633, 23.0256) ccw
  arc A526 (-9.0536, 22.4774) -> (-8.9194, 22.7243) centre (-9.7513, 23.0163) ccw
  arc A527 (-8.9194, 22.7243) -> (-8.8734, 22.9959) centre (-9.6884, 22.9943) ccw
  arc A528 (-8.8734, 22.9959) -> (-8.9614, 23.3705) centre (-9.7212, 22.9942) ccw
  arc A529 (-8.9614, 23.3705) -> (-9.2064, 23.6715) centre (-9.7465, 22.9817) ccw
  arc A530 (-9.2064, 23.6715) -> (-9.5559, 23.8357) centre (-9.7402, 22.9898) ccw
  arc A531 (-9.5559, 23.8357) -> (-9.9363, 23.8281) centre (-9.73, 23.0363) ccw
  arc A532 (-9.9363, 23.8281) -> (-10.1561, 23.7402) centre (-9.6975, 22.9113) ccw
  arc A533 (-10.1561, 23.7402) -> (-10.3382, 23.6031) centre (-9.7607, 23.0257) ccw
  arc A534 (-10.3382, 23.6031) -> (-10.4753, 23.421) centre (-9.7607, 23.0257) ccw
  arc A535 (-10.4753, 23.421) -> (-10.5631, 23.2012) centre (-9.6464, 22.9624) ccw
  arc A536 (-10.5631, 23.2012) -> (-10.5703, 22.8166) centre (-9.767, 22.9938) ccw
  arc A537 (-10.5703, 22.8166) -> (-10.4026, 22.4656) centre (-9.7328, 23.0014) ccw
  arc A538 (-10.4026, 22.4656) -> (-10.0955, 22.2227) centre (-9.7225, 23.0096) ccw
  arc A539 (-10.0955, 22.2227) -> (-9.7141, 22.1398) centre (-9.7268, 23.0004) ccw
  arc A540 (-9.7141, 22.1398) -> (-9.6642, 22.1422) centre (-9.7254, 22.9033) ccw
  arc A541 (-9.6642, 22.1422) -> (-9.6086, 22.1479) centre (-9.7604, 23.3386) ccw
  arc A542 (-9.6086, 22.1479) -> (-9.5557, 22.1559) centre (-9.7521, 23.2734) ccw
  arc A543 (-9.5557, 22.1559) -> (-9.5151, 22.1652) centre (-9.6295, 22.5755) ccw
  line L81 (-31.75, 88.9) -> (-31.75, 1)
  line L82 (-28.9873, 72.9588) -> (-29.6096, 73.5307)
  line L83 (-29.6096, 73.5307) -> (-30.2319, 74.1026)
  line L84 (-30.2319, 74.1026) -> (-30.1343, 74.2285)
  line L85 (-28.8207, 73.1484) -> (-28.9873, 72.9588)
  arc A544 (-29.9306, 74.461) -> (-30.1343, 74.2285) centre (-28.0795, 72.6342) ccw
  arc A545 (-29.5272, 74.8608) -> (-29.9306, 74.461) centre (-11.6488, 56.4197) ccw
  arc A546 (-27.8406, 74.1014) -> (-28.8207, 73.1484) centre (-22.2817, 67.4036) ccw
  arc A547 (-29.1063, 75.2589) -> (-29.5272, 74.8608) centre (-13.2395, 58.0605) ccw
  arc A548 (-28.8025, 75.5196) -> (-29.1063, 75.2589) centre (-25.3293, 71.1649) ccw
  arc A549 (-22.1093, 77.714) -> (-22.5184, 77.7217) centre (-22.5404, 65.6356) ccw
  arc A550 (-21.7493, 77.6923) -> (-22.1093, 77.714) centre (-22.3704, 70.3977) ccw
  arc A551 (-20.8534, 75.8477) -> (-21.6912, 75.9752) centre (-22.5018, 67.8321) ccw
  arc A552 (-20.7901, 74.7422) -> (-21.7493, 74.9209) centre (-22.6851, 67.236) ccw
  arc A553 (-22.5184, 77.7217) -> (-22.9286, 77.7155) centre (-22.5405, 65.582) ccw
  arc A554 (-21.6912, 75.9752) -> (-22.5501, 76.0178) centre (-22.5501, 67.3469) ccw
  arc A555 (-21.7493, 74.9209) -> (-22.0476, 74.9433) centre (-22.1391, 71.7201) ccw
  arc A556 (-22.0476, 74.9433) -> (-22.5098, 74.9502) centre (-22.5361, 57.7224) ccw
  arc A557 (-22.5501, 76.0178) -> (-23.4089, 75.9752) centre (-22.5501, 67.3469) ccw
  arc A558 (-22.9286, 77.7155) -> (-23.2925, 77.6951) centre (-22.6866, 70.1483) ccw
  arc A559 (-23.2925, 77.6951) -> (-24.788, 77.4649) centre (-22.4575, 67.2961) ccw
  arc A560 (-24.788, 77.4649) -> (-26.215, 77.0225) centre (-22.572, 67.7955) ccw
  arc A561 (-22.1959, 69.3977) -> (-22.2622, 69.4127) centre (-22.3824, 68.7282) ccw
  arc A562 (-22.2622, 69.4127) -> (-22.3484, 69.4257) centre (-22.5824, 67.5898) ccw
  arc A563 (-22.3484, 69.4257) -> (-22.4392, 69.4352) centre (-22.596, 67.4834) ccw
  arc A564 (-22.4392, 69.4352) -> (-22.5205, 69.439) centre (-22.5389, 68.1934) ccw
  arc A565 (-22.5205, 69.439) -> (-23.1428, 69.3039) centre (-22.5413, 68.0351) ccw
  arc A566 (-23.1428, 69.3039) -> (-23.6436, 68.9075) centre (-22.5342, 68.02) ccw
  arc A567 (-23.6436, 68.9075) -> (-23.9173, 68.335) centre (-22.551, 68.0335) ccw
  arc A568 (-24.517, 69.6632) -> (-24.8106, 69.3092) centre (-22.7785, 67.9227) ccw
  arc A569 (-24.8511, 69.2532) -> (-24.8106, 69.3092) centre (-25.8767, 70.0366) ccw
  arc A570 (-24.8891, 69.2074) -> (-24.8511, 69.2532) centre (-25.4156, 69.6844) ccw
  arc A571 (-19.535, 69.7486) -> (-18.9407, 70.3082) centre (-1491.7979, 1633.9609) ccw
  arc A572 (-20.1215, 69.197) -> (-19.535, 69.7486) centre (-773.3736, 870.6675) ccw
  arc A573 (-20.6547, 69.7346) -> (-21.0532, 70.05) centre (-22.5801, 67.7116) ccw
  arc A574 (-20.3253, 69.3557) -> (-20.6547, 69.7346) centre (-22.4898, 67.8065) ccw
  arc A575 (-20.3253, 69.3557) -> (-20.2704, 69.2821) centre (-18.3798, 70.7483) ccw
  arc A576 (-20.2704, 69.2821) -> (-20.2204, 69.2215) centre (-19.2538, 70.0705) ccw
  arc A577 (-20.2204, 69.2215) -> (-20.1773, 69.1742) centre (-18.9101, 70.3724) ccw
  arc A578 (-20.1773, 69.1742) -> (-20.163, 69.1709) centre (-20.1677, 69.1832) ccw
  arc A579 (-20.163, 69.1709) -> (-20.1215, 69.197) centre (-20.2086, 69.2897) ccw
  arc A580 (-22.6466, 70.4837) -> (-23.0157, 70.4561) centre (-22.4907, 65.9186) ccw
  arc A581 (-23.0157, 70.4561) -> (-23.2992, 70.399) centre (-22.8166, 68.7357) ccw
  arc A582 (-23.7319, 70.2293) -> (-24.1478, 69.9772) centre (-22.3638, 67.5029) ccw
  arc A583 (-23.2992, 70.399) -> (-23.7319, 70.2293) centre (-22.5894, 67.9526) ccw
  arc A584 (-19.2886, 70.7646) -> (-19.4784, 70.9563) centre (-24.0751, 66.2158) ccw
  arc A585 (-19.1076, 70.5661) -> (-19.2886, 70.7646) centre (-23.9951, 66.2919) ccw
  arc A586 (-18.9499, 70.3821) -> (-19.1076, 70.5661) centre (-28.4315, 62.4121) ccw
  arc A587 (-18.9311, 70.3304) -> (-18.9499, 70.3821) centre (-19.0114, 70.3304) ccw
  arc A588 (-18.9407, 70.3082) -> (-18.9311, 70.3304) centre (-18.9617, 70.3304) ccw
  arc A589 (-25.3324, 71.2088) -> (-25.71, 70.8727) centre (-21.8751, 66.9438) ccw
  arc A590 (-26.0156, 70.5345) -> (-26.0744, 70.4597) centre (-19.8293, 65.6119) ccw
  line L86 (-26.8348, 71.2147) -> (-26.9607, 71.0627)
  line L87 (-26.9607, 71.0627) -> (-27.5777, 71.6459)
  arc A591 (-18.265, 71.2144) -> (-18.7781, 71.7621) centre (-22.997, 67.2955) ccw
  line L88 (-18.1388, 71.062) -> (-18.265, 71.2144)
  line L89 (-17.5214, 71.6449) -> (-18.1388, 71.062)
  arc A592 (-19.9541, 72.611) -> (-20.6097, 72.907) centre (-22.4724, 67.9074) ccw
  arc A593 (-19.4784, 70.9563) -> (-20.0695, 71.4395) centre (-22.6192, 67.7173) ccw
  arc A594 (-18.7781, 71.7621) -> (-19.3423, 72.2287) centre (-22.6001, 67.7158) ccw
  arc A595 (-19.3423, 72.2287) -> (-19.9541, 72.611) centre (-22.5031, 67.8501) ccw
  arc A596 (-20.0695, 71.4395) -> (-20.723, 71.8059) centre (-22.436, 67.9846) ccw
  arc A597 (-22.2421, 72.1952) -> (-22.4417, 72.2028) centre (-22.405, 70.5405) ccw
  arc A598 (-21.4456, 72.0566) -> (-22.2421, 72.1952) centre (-22.7768, 66.7647) ccw
  arc A599 (-20.6097, 72.907) -> (-22.2924, 73.2541) centre (-22.5747, 67.6328) ccw
  arc A600 (-20.723, 71.8059) -> (-21.4456, 72.0566) centre (-22.5132, 67.8125) ccw
  arc A601 (-22.2768, 70.4813) -> (-22.6466, 70.4837) centre (-22.4908, 65.9221) ccw
  arc A602 (-21.0532, 70.05) -> (-21.5046, 70.2896) centre (-22.5983, 67.6837) ccw
  arc A603 (-21.5046, 70.2896) -> (-21.9913, 70.4437) centre (-22.5931, 67.6961) ccw
  arc A604 (-21.9913, 70.4437) -> (-22.2768, 70.4813) centre (-22.3569, 68.7745) ccw
  line L90 (-16.1129, 72.9581) -> (-16.2792, 73.148)
  line L91 (-15.4909, 73.5307) -> (-16.1129, 72.9581)
  arc A605 (-16.2792, 73.148) -> (-17.2547, 74.0978) centre (-22.713, 67.5159) ccw
  arc A606 (-17.2547, 74.0978) -> (-18.369, 74.8812) centre (-22.723, 67.5038) ccw
  arc A607 (-17.9264, 73.2773) -> (-18.1919, 73.4959) centre (-20.229, 70.7511) ccw
  arc A608 (-17.523, 72.8999) -> (-17.9264, 73.2773) centre (-32.0779, 57.7515) ccw
  line L92 (-16.9041, 72.2278) -> (-17.5214, 71.6449)
  line L93 (-16.9689, 72.3209) -> (-16.9041, 72.2278)
  arc A609 (-16.9689, 72.3209) -> (-17.1311, 72.515) centre (-18.1573, 71.4927) ccw
  arc A610 (-17.1311, 72.515) -> (-17.523, 72.8999) centre (-34.9294, 54.7837) ccw
  arc A611 (-24.2468, 75.8477) -> (-25.5177, 75.4722) centre (-22.6646, 68.1543) ccw
  arc A612 (-23.4089, 75.9752) -> (-24.2468, 75.8477) centre (-22.5984, 67.8321) ccw
  arc A613 (-22.5098, 74.9502) -> (-22.9762, 74.9445) centre (-22.5358, 57.9715) ccw
  arc A614 (-22.9762, 74.9445) -> (-23.2982, 74.9233) centre (-22.871, 70.891) ccw
  arc A615 (-23.2982, 74.9233) -> (-23.8995, 74.8329) centre (-22.5661, 68.0123) ccw
  arc A616 (-22.2924, 73.2541) -> (-23.9835, 73.0714) centre (-22.5639, 67.8491) ccw
  arc A617 (-22.4417, 72.2028) -> (-22.7501, 72.1906) centre (-22.2458, 63.3377) ccw
  arc A618 (-24.5014, 74.689) -> (-25.0885, 74.496) centre (-22.4747, 67.5365) ccw
  arc A619 (-23.8995, 74.8329) -> (-24.5014, 74.689) centre (-22.4694, 67.518) ccw
  arc A620 (-19.0156, 74.0314) -> (-19.8802, 74.4466) centre (-22.5564, 67.7656) ccw
  arc A621 (-18.1919, 73.4959) -> (-19.0156, 74.0314) centre (-22.9131, 67.1344) ccw
  arc A622 (-19.8802, 74.4466) -> (-20.7901, 74.7422) centre (-22.543, 67.7992) ccw
  arc A623 (-18.369, 74.8812) -> (-19.5826, 75.4717) centre (-22.6425, 67.6403) ccw
  arc A624 (-18.6997, 76.949) -> (-20.187, 77.4376) centre (-22.5214, 67.8245) ccw
  arc A625 (-17.3094, 76.2324) -> (-18.6997, 76.949) centre (-22.5142, 67.8418) ccw
  arc A626 (-19.5826, 75.4717) -> (-20.8534, 75.8477) centre (-22.4288, 68.1871) ccw
  arc A627 (-20.187, 77.4376) -> (-21.7493, 77.6923) centre (-22.6264, 67.3919) ccw
  line L94 (-14.8688, 74.1034) -> (-15.4909, 73.5307)
  line L95 (-14.9627, 74.2218) -> (-14.8688, 74.1034)
  arc A628 (-14.9627, 74.2218) -> (-15.1505, 74.4393) centre (-17.6104, 72.1248) ccw
  arc A629 (-15.1505, 74.4393) -> (-15.443, 74.7415) centre (-25.9195, 64.3064) ccw
  arc A630 (-15.443, 74.7415) -> (-15.7596, 75.0502) centre (-26.1767, 64.0502) ccw
  arc A631 (-15.7596, 75.0502) -> (-16.0359, 75.2993) centre (-21.006, 69.5101) ccw
  arc A632 (-16.0359, 75.2993) -> (-17.3094, 76.2324) centre (-22.7114, 67.5238) ccw
  arc A633 (-24.9244, 71.5096) -> (-25.3324, 71.2088) centre (-21.859, 66.9241) ccw
  arc A634 (-24.5269, 71.7413) -> (-24.9244, 71.5096) centre (-22.8398, 68.3913) ccw
  arc A635 (-24.2711, 71.8543) -> (-24.5269, 71.7413) centre (-23.2821, 69.2696) ccw
  arc A636 (-23.9835, 73.0714) -> (-25.5409, 72.3712) centre (-22.5518, 67.8045) ccw
  arc A637 (-23.9386, 71.9719) -> (-24.2711, 71.8543) centre (-21.8001, 65.3962) ccw
  arc A638 (-23.5989, 72.0729) -> (-23.9386, 71.9719) centre (-21.7906, 65.3668) ccw
  arc A639 (-23.3201, 72.1338) -> (-23.5989, 72.0729) centre (-22.8297, 69.2201) ccw
  arc A640 (-23.0696, 72.1665) -> (-23.3201, 72.1338) centre (-22.7486, 68.7389) ccw
  arc A641 (-24.1478, 69.9772) -> (-24.517, 69.6632) centre (-22.3756, 67.5193) ccw
  arc A642 (-22.7501, 72.1906) -> (-23.0696, 72.1665) centre (-22.2504, 63.417) ccw
  arc A643 (-26.215, 77.0225) -> (-27.5579, 76.3713) centre (-22.5806, 67.8172) ccw
  arc A644 (-26.206, 73.9616) -> (-26.7098, 73.6373) centre (-22.9574, 68.3625) ccw
  arc A645 (-26.728, 74.8838) -> (-27.8406, 74.1014) centre (-22.3923, 67.5369) ccw
  arc A646 (-25.6455, 74.2582) -> (-26.206, 73.9616) centre (-22.1302, 66.9368) ccw
  arc A647 (-27.5579, 76.3713) -> (-28.8025, 75.5196) centre (-22.3681, 67.4521) ccw
  arc A648 (-25.0885, 74.496) -> (-25.6455, 74.2582) centre (-22.6775, 68.0766) ccw
  arc A649 (-25.5177, 75.4722) -> (-26.728, 74.8838) centre (-22.4854, 67.6947) ccw
  arc A650 (-26.7098, 73.6373) -> (-27.1822, 73.2672) centre (-22.9439, 68.3435) ccw
  arc A651 (-27.1822, 73.2672) -> (-27.6487, 72.8332) centre (-21.8003, 67.0149) ccw
  arc A652 (-27.6487, 72.8332) -> (-27.8131, 72.6659) centre (-13.9293, 59.1844) ccw
  arc A653 (-27.8131, 72.6659) -> (-27.9621, 72.51) centre (-17.8787, 63.0194) ccw
  arc A654 (-25.71, 70.8727) -> (-26.0156, 70.5345) centre (-23.1687, 68.2691) ccw
  arc A655 (-26.124, 70.3946) -> (-26.1662, 70.3377) centre (-16.1708, 62.9655) ccw
  arc A656 (-26.1662, 70.3377) -> (-26.1691, 70.3289) centre (-26.1543, 70.3289) ccw
  arc A657 (-26.1691, 70.3289) -> (-26.1598, 70.3074) centre (-26.1396, 70.3289) ccw
  arc A658 (-26.1598, 70.3074) -> (-25.5642, 69.7477) centre (1546.327, 1742.9056) ccw
  arc A659 (-25.5642, 69.7477) -> (-24.9763, 69.1957) centre (786.502, 934.1296) ccw
  arc A660 (-24.9763, 69.1957) -> (-24.9361, 69.1706) centre (-24.8925, 69.285) ccw
  arc A661 (-24.9361, 69.1706) -> (-24.9219, 69.1735) centre (-24.9313, 69.1832) ccw
  arc A662 (-24.9219, 69.1735) -> (-24.8891, 69.2074) centre (-25.425, 69.6929) ccw
  arc A663 (-27.9621, 72.51) -> (-28.0852, 72.3777) centre (-16.9966, 62.1891) ccw
  arc A664 (-28.0852, 72.3777) -> (-28.1302, 72.3216) centre (-27.6891, 72.0138) ccw
  line L96 (-28.1947, 72.2292) -> (-28.1302, 72.3216)
  line L97 (-27.5777, 71.6459) -> (-28.1947, 72.2292)
  arc A665 (-25.5409, 72.3712) -> (-26.8348, 71.2147) centre (-22.3565, 67.5061) ccw
  arc A666 (-26.0744, 70.4597) -> (-26.124, 70.3946) centre (-22.6541, 67.8046) ccw
  arc A667 (-21.7797, 69.2048) -> (-22.1959, 69.3977) centre (-22.5776, 68.0282) ccw
  arc A668 (-21.443, 68.8883) -> (-21.7797, 69.2048) centre (-22.6008, 67.9939) ccw
  arc A669 (-21.2241, 68.4855) -> (-21.443, 68.8883) centre (-22.5811, 68.0091) ccw
  arc A670 (-21.149, 68.0425) -> (-21.2241, 68.4855) centre (-22.4786, 68.0451) ccw
  arc A671 (-21.2927, 67.4314) -> (-21.149, 68.0425) centre (-22.5322, 68.0452) ccw
  arc A672 (-22.8829, 66.6849) -> (-22.2625, 66.6724) centre (-22.5465, 67.9765) ccw
  arc A673 (-23.2415, 66.8282) -> (-22.8829, 66.6849) centre (-22.4934, 68.1804) ccw
  arc A674 (-23.9173, 68.335) -> (-23.9055, 67.7075) centre (-22.6068, 68.0458) ccw
  arc A675 (-23.5386, 67.0519) -> (-23.2415, 66.8282) centre (-22.5966, 67.9939) ccw
  arc A676 (-23.7623, 67.3489) -> (-23.5386, 67.0519) centre (-22.5966, 67.9939) ccw
  arc A677 (-23.9055, 67.7075) -> (-23.7623, 67.3489) centre (-22.4101, 68.0971) ccw
  arc A678 (-22.2625, 66.6724) -> (-21.6924, 66.9404) centre (-22.563, 68.0524) ccw
  arc A679 (-21.6924, 66.9404) -> (-21.2927, 67.4314) centre (-22.5734, 68.0656) ccw
  line L98 (-34.5127, 15.9412) -> (-33.8904, 15.3693)
  line L99 (-33.8904, 15.3693) -> (-33.2681, 14.7974)
  line L100 (-33.2681, 14.7974) -> (-33.3657, 14.6715)
  line L101 (-34.6793, 15.7516) -> (-34.5127, 15.9412)
  arc A680 (-33.5694, 14.439) -> (-33.3657, 14.6715) centre (-35.4205, 16.2658) ccw
  arc A681 (-33.9728, 14.0392) -> (-33.5694, 14.439) centre (-51.8512, 32.4803) ccw
  arc A682 (-35.6594, 14.7986) -> (-34.6793, 15.7516) centre (-41.2183, 21.4964) ccw
  arc A683 (-34.3937, 13.6411) -> (-33.9728, 14.0392) centre (-50.2605, 30.8395) ccw
  arc A684 (-34.6975, 13.3804) -> (-34.3937, 13.6411) centre (-38.1707, 17.7351) ccw
  arc A685 (-41.3907, 11.186) -> (-40.9816, 11.1783) centre (-40.9596, 23.2644) ccw
  arc A686 (-41.7507, 11.2077) -> (-41.3907, 11.186) centre (-41.1296, 18.5023) ccw
  arc A687 (-42.6466, 13.0523) -> (-41.8088, 12.9248) centre (-40.9982, 21.0679) ccw
  arc A688 (-42.7099, 14.1578) -> (-41.7507, 13.9791) centre (-40.8149, 21.664) ccw
  arc A689 (-40.9816, 11.1783) -> (-40.5714, 11.1845) centre (-40.9595, 23.318) ccw
  arc A690 (-41.8088, 12.9248) -> (-40.9499, 12.8822) centre (-40.9499, 21.5531) ccw
  arc A691 (-41.7507, 13.9791) -> (-41.4524, 13.9567) centre (-41.3609, 17.1799) ccw
  arc A692 (-41.4524, 13.9567) -> (-40.9902, 13.9498) centre (-40.9639, 31.1776) ccw
  arc A693 (-40.9499, 12.8822) -> (-40.0911, 12.9248) centre (-40.9499, 21.5531) ccw
  arc A694 (-40.5714, 11.1845) -> (-40.2075, 11.2049) centre (-40.8134, 18.7517) ccw
  arc A695 (-40.2075, 11.2049) -> (-38.712, 11.4351) centre (-41.0425, 21.6039) ccw
  arc A696 (-38.712, 11.4351) -> (-37.285, 11.8775) centre (-40.928, 21.1045) ccw
  arc A697 (-41.3041, 19.5023) -> (-41.2378, 19.4873) centre (-41.1176, 20.1718) ccw
  arc A698 (-41.2378, 19.4873) -> (-41.1516, 19.4743) centre (-40.9176, 21.3102) ccw
  arc A699 (-41.1516, 19.4743) -> (-41.0608, 19.4648) centre (-40.904, 21.4166) ccw
  arc A700 (-41.0608, 19.4648) -> (-40.9795, 19.461) centre (-40.9611, 20.7066) ccw
  arc A701 (-40.9795, 19.461) -> (-40.3572, 19.5961) centre (-40.9587, 20.8649) ccw
  arc A702 (-40.3572, 19.5961) -> (-39.8564, 19.9925) centre (-40.9658, 20.88) ccw
  arc A703 (-39.8564, 19.9925) -> (-39.5827, 20.565) centre (-40.949, 20.8665) ccw
  arc A704 (-38.983, 19.2368) -> (-38.6894, 19.5908) centre (-40.7215, 20.9773) ccw
  arc A705 (-38.6489, 19.6468) -> (-38.6894, 19.5908) centre (-37.6233, 18.8634) ccw
  arc A706 (-38.6109, 19.6926) -> (-38.6489, 19.6468) centre (-38.0844, 19.2156) ccw
  arc A707 (-43.965, 19.1514) -> (-44.5593, 18.5918) centre (1428.2979, -1545.0609) ccw
  arc A708 (-43.3785, 19.703) -> (-43.965, 19.1514) centre (709.8736, -781.7675) ccw
  arc A709 (-42.8453, 19.1654) -> (-42.4468, 18.85) centre (-40.9199, 21.1884) ccw
  arc A710 (-43.1747, 19.5443) -> (-42.8453, 19.1654) centre (-41.0102, 21.0935) ccw
  arc A711 (-43.1747, 19.5443) -> (-43.2296, 19.6179) centre (-45.1202, 18.1517) ccw
  arc A712 (-43.2296, 19.6179) -> (-43.2796, 19.6785) centre (-44.2462, 18.8295) ccw
  arc A713 (-43.2796, 19.6785) -> (-43.3227, 19.7258) centre (-44.5899, 18.5276) ccw
  arc A714 (-43.3227, 19.7258) -> (-43.337, 19.7291) centre (-43.3323, 19.7168) ccw
  arc A715 (-43.337, 19.7291) -> (-43.3785, 19.703) centre (-43.2914, 19.6103) ccw
  arc A716 (-40.8534, 18.4163) -> (-40.4843, 18.4439) centre (-41.0093, 22.9814) ccw
  arc A717 (-40.4843, 18.4439) -> (-40.2008, 18.501) centre (-40.6834, 20.1643) ccw
  arc A718 (-39.7681, 18.6707) -> (-39.3522, 18.9228) centre (-41.1362, 21.3971) ccw
  arc A719 (-40.2008, 18.501) -> (-39.7681, 18.6707) centre (-40.9106, 20.9474) ccw
  arc A720 (-44.2114, 18.1354) -> (-44.0216, 17.9437) centre (-39.4249, 22.6842) ccw
  arc A721 (-44.3924, 18.3339) -> (-44.2114, 18.1354) centre (-39.5049, 22.6081) ccw
  arc A722 (-44.5501, 18.5179) -> (-44.3924, 18.3339) centre (-35.0685, 26.4879) ccw
  arc A723 (-44.5689, 18.5696) -> (-44.5501, 18.5179) centre (-44.4886, 18.5696) ccw
  arc A724 (-44.5593, 18.5918) -> (-44.5689, 18.5696) centre (-44.5383, 18.5696) ccw
  arc A725 (-38.1676, 17.6912) -> (-37.79, 18.0273) centre (-41.6249, 21.9562) ccw
  arc A726 (-37.4844, 18.3655) -> (-37.4256, 18.4403) centre (-43.6707, 23.2881) ccw
  line L102 (-36.6652, 17.6853) -> (-36.5393, 17.8373)
  line L103 (-36.5393, 17.8373) -> (-35.9223, 17.2541)
  arc A727 (-45.235, 17.6856) -> (-44.7219, 17.1379) centre (-40.503, 21.6045) ccw
  line L104 (-45.3612, 17.838) -> (-45.235, 17.6856)
  line L105 (-45.9786, 17.2551) -> (-45.3612, 17.838)